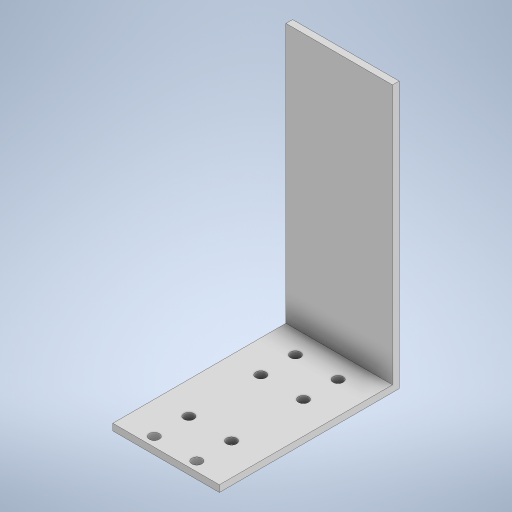
# Autodesk Inventor part: Gripper Slider Connecting Plate & Bar
Saved by Autodesk Inventor 2023 (Build 270158000, 158)
## iProperties
Created: 2023-01-18
Part Number: Gripper Slider Connecting Plate & Bar
Material: Generic
Document SubType Name: Modeling
Designer: Gabriel - T3 CAD
Density: 1 g/cm^3
Appearance: Default
Author: Gabriel - T3 CAD
Autodesk Inventor part; units mm, degrees
ref_plane "YZ Plane" through (0, 0, 0) normal (1, 0, 0) x (0, 1, 0)
ref_plane "XZ Plane" through (0, 0, 0) normal (0, 1, 0) x (-1, 0, 0)
ref_plane "XY Plane" through (0, 0, 0) normal (0, 0, 1) x (1, 0, 0)
sketch "Sketch1" plane through (0, 0, 0) normal (0, 1, 0) x (-1, 0, 0)
  line L0 (0, 0) -> (50.8, 0)
  line L1 (50.8, 0) -> (50.8, 76.2)
  line L2 (50.8, 76.2) -> (0, 76.2)
  line L3 (0, 76.2) -> (0, 0)
  circle A0 centre (35.4838, 71.755) radius 2.3813
  circle A1 centre (35.4838, 55.245) radius 2.3813
  circle A2 centre (15.1638, 71.755) radius 2.3813
  circle A3 centre (15.1638, 55.245) radius 2.3813
  line L4 (50.8, 38.1) -> (0, 38.1)
  circle A4 centre (35.4838, 4.445) radius 2.3813
  circle A5 centre (35.4838, 20.955) radius 2.3813
  circle A6 centre (15.1638, 4.445) radius 2.3813
  circle A7 centre (15.1638, 20.955) radius 2.3813
  line L5 (0, 0) -> (50.8, 0)
  line L6 (50.8, 0) -> (50.8, -6.35)
  line L7 (50.8, -6.35) -> (0, -6.35)
  line L8 (0, -6.35) -> (0, 0)
  line L9 (0, -6.35) -> (50.8, -6.35)
  line L10 (50.8, -6.35) -> (50.8, -9.525)
  line L11 (50.8, -9.525) -> (0, -9.525)
  line L12 (0, -9.525) -> (0, -6.35)
  dimension "d0" = 50.8
  dimension "d1" = 76.2
  dimension "d2" = 4.7625
  dimension "d3" = 15.3162
  dimension "d4" = 4.445
  dimension "d7" = 16.51
  dimension "d10" = 20.32
  dimension "d15" = 50.8
  dimension "d16" = 6.35
  dimension "d17" = 50.8
  dimension "d18" = 3.175
  constraints: 26 end point, 8 centre point, 6 parallel, 4 horizontal, 4 symmetric about line, 3 perpendicular, 2 midpoint, 1 vertical, 10 other
  measures "d0" distance of L2.end L1.end
  measures "d1" distance of L1.end L0.end
  measures "d2" diameter of A0
  measures "d3" distance from line of L1 A0.centre
  measures "d4" distance from line of L2 A0.centre
  measures "d7" distance of A0.centre A1.centre
  measures "d10" distance of A0.centre A2.centre
  measures "d15" distance of L6.end L7.end
  measures "d16" distance of L5.end L6.end
  measures "d17" distance of L10.end L11.end
  measures "d18" distance of L9.end L10.end
extrude "Extrusion1" add sketch "Sketch1" along normal blind 3.175
extrude "Extrusion2" add sketch "Sketch1" along normal blind 127 contours L7 L10 L11 L12
body "Solid1"
